Autodesk Inventor part; units mm, degrees
(part 2 of 2)
  spline S28 degree 3 poles (-3.689, -11.9815) (-3.6809, -11.9574) (-3.6638, -11.908) (-3.6373, -11.8352) (-3.6101, -11.7647) (-3.5836, -11.699) (-3.5531, -11.629) (-3.5301, -11.5735) (-3.5094, -11.5336) (-3.5004, -11.5147) (-3.492, -11.4959) (-3.4842, -11.4771) (-3.477, -11.4583) (-3.4704, -11.4394) (-3.4644, -11.4203) (-3.4591, -11.401) (-3.4546, -11.3811) (-3.4508, -11.3607) (-3.4479, -11.3394) (-3.4461, -11.3171) (-3.4456, -11.2935) (-3.4468, -11.2683) (-3.4503, -11.2414) (-3.4567, -11.2125) (-3.4668, -11.1819) (-3.4815, -11.1502) (-3.5016, -11.1183) (-3.5261, -11.0891) (-3.5749, -11.0459) (-3.6488, -10.9917) (-3.7179, -10.9316) (-3.7709, -10.8935) (-3.8047, -10.876) (-3.8402, -10.8634) (-3.8745, -10.8561) (-3.9066, -10.853) (-3.9361, -10.8531) (-3.9632, -10.8557) (-3.988, -10.86) (-4.0109, -10.8657) (-4.0323, -10.8724) (-4.0524, -10.8799) (-4.0715, -10.8881) (-4.0898, -10.8969) (-4.1075, -10.9063) (-4.1248, -10.9164) (-4.1418, -10.9269) (-4.1585, -10.9381) (-4.1751, -10.9499) (-4.1916, -10.9622) (-4.2081, -10.9752) (-4.2425, -11.0042) (-4.2915, -11.0389) (-4.3531, -11.084) (-4.4113, -11.1243) (-4.4741, -11.1664) (-4.5392, -11.2083) (-4.5836, -11.2358) (-4.6054, -11.2491) knots 0 0 0 0 0.034227 0.070321 0.104238 0.13598 0.165545 0.207076 0.216654 0.226052 0.235294 0.244406 0.25342 0.262376 0.27132 0.280307 0.289405 0.298694 0.308273 0.31826 0.328793 0.340032 0.352153 0.365336 0.379732 0.395424 0.412362 0.430317 0.446471 0.5 0.553529 0.569683 0.587638 0.604576 0.620268 0.634664 0.647847 0.659968 0.671207 0.68174 0.691727 0.701306 0.710595 0.719693 0.72868 0.737624 0.74658 0.755594 0.764706 0.773948 0.783346 0.792924 0.834455 0.86402 0.895762 0.929679 0.965773 1 1 1 1
  arc A28 (-3.689, -11.9815) -> (-2.6062, -12.7155) centre (5.7104, 0.7186) ccw
  spline S29 degree 3 poles (-1.5865, -13.2955) (-1.5823, -13.2704) (-1.5731, -13.219) (-1.5583, -13.1429) (-1.5425, -13.069) (-1.5266, -13) (-1.5075, -12.9261) (-1.4934, -12.8677) (-1.4792, -12.8251) (-1.4733, -12.805) (-1.4679, -12.785) (-1.4631, -12.7653) (-1.459, -12.7456) (-1.4554, -12.7259) (-1.4525, -12.7061) (-1.4503, -12.6862) (-1.4489, -12.6659) (-1.4483, -12.6451) (-1.4488, -12.6236) (-1.4505, -12.6013) (-1.4538, -12.5779) (-1.4589, -12.5533) (-1.4666, -12.5272) (-1.4774, -12.4997) (-1.4921, -12.4711) (-1.5116, -12.442) (-1.5365, -12.4136) (-1.5653, -12.3887) (-1.6202, -12.3536) (-1.7017, -12.3116) (-1.7794, -12.263) (-1.8376, -12.2337) (-1.8738, -12.2217) (-1.9108, -12.2149) (-1.9458, -12.213) (-1.978, -12.2149) (-2.0071, -12.2197) (-2.0334, -12.2265) (-2.0573, -12.2346) (-2.0791, -12.2438) (-2.0991, -12.2537) (-2.1178, -12.2643) (-2.1354, -12.2754) (-2.1521, -12.287) (-2.1681, -12.2991) (-2.1836, -12.3117) (-2.1987, -12.3248) (-2.2135, -12.3384) (-2.2281, -12.3526) (-2.2424, -12.3674) (-2.2567, -12.3828) (-2.2861, -12.4168) (-2.3291, -12.4587) (-2.3829, -12.513) (-2.434, -12.5619) (-2.4895, -12.6133) (-2.5473, -12.6649) (-2.5868, -12.699) (-2.6062, -12.7155) knots 0 0 0 0 0.034227 0.070321 0.104238 0.13598 0.165545 0.207076 0.216654 0.226052 0.235294 0.244406 0.25342 0.262376 0.27132 0.280307 0.289405 0.298694 0.308273 0.31826 0.328793 0.340032 0.352153 0.365336 0.379732 0.395424 0.412362 0.430317 0.446471 0.5 0.553529 0.569683 0.587638 0.604576 0.620268 0.634664 0.647847 0.659968 0.671207 0.68174 0.691727 0.701306 0.710595 0.719693 0.72868 0.737624 0.74658 0.755594 0.764706 0.773948 0.783346 0.792924 0.834455 0.86402 0.895762 0.929679 0.965773 1 1 1 1
  arc A29 (-1.5865, -13.2955) -> (-0.4023, -13.8511) centre (5.7104, 0.7186) ccw
  spline S30 degree 3 poles (0.6956, -14.2644) (0.6959, -14.239) (0.6968, -14.1868) (0.6996, -14.1094) (0.7036, -14.0339) (0.7085, -13.9633) (0.7159, -13.8872) (0.7206, -13.8274) (0.728, -13.783) (0.7307, -13.7622) (0.7329, -13.7417) (0.7345, -13.7215) (0.7356, -13.7014) (0.736, -13.6814) (0.7358, -13.6614) (0.7348, -13.6413) (0.733, -13.621) (0.7303, -13.6004) (0.7265, -13.5793) (0.7213, -13.5576) (0.7145, -13.535) (0.7055, -13.5114) (0.6939, -13.4868) (0.6789, -13.4614) (0.6599, -13.4354) (0.6361, -13.4097) (0.6071, -13.3856) (0.5748, -13.3655) (0.515, -13.3394) (0.428, -13.3107) (0.3436, -13.2749) (0.2815, -13.255) (0.2439, -13.2488) (0.2062, -13.2479) (0.1714, -13.2515) (0.1399, -13.2584) (0.1119, -13.2677) (0.0869, -13.2785) (0.0647, -13.2903) (0.0446, -13.3028) (0.0264, -13.3157) (0.0096, -13.3291) (-0.006, -13.3428) (-0.0207, -13.3568) (-0.0347, -13.3713) (-0.048, -13.3861) (-0.0609, -13.4015) (-0.0734, -13.4173) (-0.0855, -13.4336) (-0.0974, -13.4504) (-0.1091, -13.4678) (-0.1328, -13.506) (-0.1687, -13.5542) (-0.2133, -13.6161) (-0.2562, -13.6724) (-0.303, -13.7319) (-0.352, -13.7919) (-0.3857, -13.8318) (-0.4023, -13.8511) knots 0 0 0 0 0.034227 0.070321 0.104238 0.13598 0.165545 0.207076 0.216654 0.226052 0.235294 0.244406 0.25342 0.262376 0.27132 0.280307 0.289405 0.298694 0.308273 0.31826 0.328793 0.340032 0.352153 0.365336 0.379732 0.395424 0.412362 0.430317 0.446471 0.5 0.553529 0.569683 0.587638 0.604576 0.620268 0.634664 0.647847 0.659968 0.671207 0.68174 0.691727 0.701306 0.710595 0.719693 0.72868 0.737624 0.74658 0.755594 0.764706 0.773948 0.783346 0.792924 0.834455 0.86402 0.895762 0.929679 0.965773 1 1 1 1
  arc A30 (0.6956, -14.2644) -> (1.9522, -14.6279) centre (5.7104, 0.7186) ccw
  spline S31 degree 3 poles (3.1012, -14.8645) (3.0975, -14.8393) (3.0903, -14.7875) (3.0809, -14.7107) (3.0731, -14.6355) (3.0669, -14.565) (3.0622, -14.4887) (3.0576, -14.4289) (3.0579, -14.3839) (3.0573, -14.3629) (3.0563, -14.3423) (3.0547, -14.3221) (3.0526, -14.3021) (3.0499, -14.2822) (3.0465, -14.2625) (3.0425, -14.2429) (3.0375, -14.2231) (3.0316, -14.2032) (3.0246, -14.1829) (3.016, -14.1623) (3.0057, -14.141) (2.9932, -14.1191) (2.9779, -14.0967) (2.9591, -14.0739) (2.9362, -14.0512) (2.9087, -14.0296) (2.8763, -14.0103) (2.8412, -13.9955) (2.7781, -13.979) (2.6877, -13.9643) (2.5988, -13.9421) (2.5343, -13.9323) (2.4962, -13.932) (2.4589, -13.937) (2.425, -13.946) (2.395, -13.9577) (2.3688, -13.9713) (2.3458, -13.9859) (2.3257, -14.001) (2.3078, -14.0165) (2.2918, -14.0321) (2.2773, -14.0479) (2.264, -14.0639) (2.2517, -14.0801) (2.2402, -14.0965) (2.2293, -14.1133) (2.219, -14.1304) (2.2092, -14.148) (2.1997, -14.166) (2.1906, -14.1845) (2.1818, -14.2035) (2.1644, -14.245) (2.1364, -14.2981) (2.102, -14.3663) (2.0685, -14.4286) (2.0316, -14.4947) (1.9926, -14.5616) (1.9655, -14.6063) (1.9522, -14.6279) knots 0 0 0 0 0.034227 0.070321 0.104238 0.13598 0.165545 0.207076 0.216654 0.226052 0.235294 0.244406 0.25342 0.262376 0.27132 0.280307 0.289405 0.298694 0.308273 0.31826 0.328793 0.340032 0.352153 0.365336 0.379732 0.395424 0.412362 0.430317 0.446471 0.5 0.553529 0.569683 0.587638 0.604576 0.620268 0.634664 0.647847 0.659968 0.671207 0.68174 0.691727 0.701306 0.710595 0.719693 0.72868 0.737624 0.74658 0.755594 0.764706 0.773948 0.783346 0.792924 0.834455 0.86402 0.895762 0.929679 0.965773 1 1 1 1
  arc A31 (3.1012, -14.8645) -> (4.3992, -15.0269) centre (5.7104, 0.7186) ccw
  spline S32 degree 3 poles (5.5711, -15.0808) (5.5635, -15.0565) (5.5482, -15.0065) (5.5269, -14.932) (5.5075, -14.859) (5.4903, -14.7903) (5.4738, -14.7157) (5.4598, -14.6574) (5.4531, -14.6129) (5.4493, -14.5923) (5.445, -14.5721) (5.4403, -14.5523) (5.4351, -14.5329) (5.4293, -14.5137) (5.4229, -14.4948) (5.4158, -14.476) (5.4079, -14.4573) (5.3989, -14.4385) (5.3888, -14.4196) (5.3771, -14.4005) (5.3636, -14.3812) (5.3478, -14.3615) (5.3292, -14.3417) (5.307, -14.3221) (5.2809, -14.3033) (5.2503, -14.2863) (5.2153, -14.2723) (5.1783, -14.2631) (5.1134, -14.2568) (5.0218, -14.2564) (4.9305, -14.2484) (4.8653, -14.2487) (4.8277, -14.2545) (4.7915, -14.2652) (4.7595, -14.2794) (4.7317, -14.2957) (4.7079, -14.3132) (4.6875, -14.3312) (4.67, -14.3493) (4.6548, -14.3673) (4.6414, -14.3853) (4.6296, -14.4032) (4.6189, -14.421) (4.6093, -14.4389) (4.6005, -14.457) (4.5924, -14.4753) (4.5849, -14.4938) (4.5779, -14.5127) (4.5714, -14.5319) (4.5653, -14.5517) (4.5596, -14.5718) (4.5488, -14.6155) (4.5296, -14.6723) (4.5063, -14.7451) (4.4829, -14.8119) (4.4568, -14.8828) (4.4287, -14.955) (4.409, -15.0034) (4.3992, -15.0269) knots 0 0 0 0 0.034227 0.070321 0.104238 0.13598 0.165545 0.207076 0.216654 0.226052 0.235294 0.244406 0.25342 0.262376 0.27132 0.280307 0.289405 0.298694 0.308273 0.31826 0.328793 0.340032 0.352153 0.365336 0.379732 0.395424 0.412362 0.430317 0.446471 0.5 0.553529 0.569683 0.587638 0.604576 0.620268 0.634664 0.647847 0.659968 0.671207 0.68174 0.691727 0.701306 0.710595 0.719693 0.72868 0.737624 0.74658 0.755594 0.764706 0.773948 0.783346 0.792924 0.834455 0.86402 0.895762 0.929679 0.965773 1 1 1 1
  arc A32 (5.5711, -15.0808) -> (6.8785, -15.0381) centre (5.7104, 0.7186) ccw
  spline S33 degree 3 poles (8.0444, -14.908) (8.0331, -14.8853) (8.0102, -14.8383) (7.9775, -14.7681) (7.9468, -14.6989) (7.9192, -14.6338) (7.8912, -14.5627) (7.8682, -14.5073) (7.8547, -14.4644) (7.8476, -14.4446) (7.8403, -14.4254) (7.8325, -14.4066) (7.8243, -14.3882) (7.8156, -14.3702) (7.8064, -14.3525) (7.7964, -14.335) (7.7856, -14.3178) (7.7738, -14.3006) (7.7609, -14.2836) (7.7464, -14.2665) (7.73, -14.2495) (7.7113, -14.2326) (7.6898, -14.216) (7.6649, -14.2001) (7.6361, -14.1856) (7.6033, -14.1735) (7.5665, -14.1652) (7.5285, -14.1619) (7.4634, -14.1658) (7.3729, -14.1798) (7.2815, -14.1861) (7.2171, -14.1967) (7.1808, -14.2082) (7.1468, -14.2244) (7.1174, -14.2435) (7.0925, -14.2639) (7.0717, -14.2849) (7.0544, -14.3059) (7.0399, -14.3265) (7.0277, -14.3467) (7.0173, -14.3665) (7.0084, -14.3861) (7.0007, -14.4054) (6.994, -14.4246) (6.9882, -14.4438) (6.983, -14.4631) (6.9785, -14.4826) (6.9746, -14.5023) (6.9711, -14.5224) (6.9682, -14.5428) (6.9657, -14.5636) (6.9619, -14.6084) (6.9518, -14.6676) (6.9402, -14.7431) (6.9275, -14.8127) (6.9129, -14.8869) (6.8964, -14.9626) (6.8845, -15.0134) (6.8785, -15.0381) knots 0 0 0 0 0.034227 0.070321 0.104238 0.13598 0.165545 0.207076 0.216654 0.226052 0.235294 0.244406 0.25342 0.262376 0.27132 0.280307 0.289405 0.298694 0.308273 0.31826 0.328793 0.340032 0.352153 0.365336 0.379732 0.395424 0.412362 0.430317 0.446471 0.5 0.553529 0.569683 0.587638 0.604576 0.620268 0.634664 0.647847 0.659968 0.671207 0.68174 0.691727 0.701306 0.710595 0.719693 0.72868 0.737624 0.74658 0.755594 0.764706 0.773948 0.783346 0.792924 0.834455 0.86402 0.895762 0.929679 0.965773 1 1 1 1
  arc A33 (8.0444, -14.908) -> (9.329, -14.6614) centre (5.7104, 0.7186) ccw
  spline S34 degree 3 poles (10.4602, -14.3505) (10.4454, -14.3298) (10.4155, -14.287) (10.3722, -14.2227) (10.3311, -14.1593) (10.2936, -14.0993) (10.2548, -14.0334) (10.2235, -13.9823) (10.2034, -13.942) (10.1934, -13.9236) (10.1831, -13.9057) (10.1725, -13.8884) (10.1615, -13.8715) (10.1501, -13.8551) (10.1382, -13.839) (10.1256, -13.8234) (10.1123, -13.808) (10.098, -13.7929) (10.0825, -13.7781) (10.0655, -13.7635) (10.0467, -13.7493) (10.0256, -13.7355) (10.0017, -13.7224) (9.9746, -13.7106) (9.944, -13.7008) (9.9096, -13.6941) (9.872, -13.6916) (9.834, -13.6943) (9.7703, -13.7083) (9.683, -13.7363) (9.5938, -13.7568) (9.5318, -13.7773) (9.4978, -13.7944) (9.4667, -13.8158) (9.4407, -13.8391) (9.4193, -13.8633) (9.4021, -13.8872) (9.3882, -13.9106) (9.3771, -13.9333) (9.3682, -13.9552) (9.3611, -13.9764) (9.3554, -13.997) (9.3508, -14.0173) (9.3471, -14.0373) (9.3444, -14.0572) (9.3423, -14.0771) (9.3409, -14.097) (9.3401, -14.1172) (9.3398, -14.1375) (9.3401, -14.1581) (9.3409, -14.1791) (9.3442, -14.2239) (9.3434, -14.2839) (9.3438, -14.3603) (9.3422, -14.4311) (9.3393, -14.5066) (9.3349, -14.584) (9.3311, -14.6361) (9.329, -14.6614) knots 0 0 0 0 0.034227 0.070321 0.104238 0.13598 0.165545 0.207076 0.216654 0.226052 0.235294 0.244406 0.25342 0.262376 0.27132 0.280307 0.289405 0.298694 0.308273 0.31826 0.328793 0.340032 0.352153 0.365336 0.379732 0.395424 0.412362 0.430317 0.446471 0.5 0.553529 0.569683 0.587638 0.604576 0.620268 0.634664 0.647847 0.659968 0.671207 0.68174 0.691727 0.701306 0.710595 0.719693 0.72868 0.737624 0.74658 0.755594 0.764706 0.773948 0.783346 0.792924 0.834455 0.86402 0.895762 0.929679 0.965773 1 1 1 1
  arc A34 (10.4602, -14.3505) -> (11.6904, -13.906) centre (5.7104, 0.7186) ccw
  spline S35 degree 3 poles (12.759, -13.422) (12.7412, -13.4038) (12.705, -13.3662) (12.6522, -13.3095) (12.6017, -13.2533) (12.5552, -13.1999) (12.5066, -13.1409) (12.4677, -13.0952) (12.4415, -13.0587) (12.4287, -13.0421) (12.4158, -13.026) (12.4026, -13.0105) (12.3891, -12.9956) (12.3753, -12.9811) (12.361, -12.9672) (12.3461, -12.9536) (12.3306, -12.9406) (12.3141, -12.9279) (12.2964, -12.9157) (12.2774, -12.9039) (12.2566, -12.8928) (12.2336, -12.8825) (12.208, -12.8733) (12.1794, -12.8659) (12.1475, -12.861) (12.1125, -12.8597) (12.075, -12.8631) (12.0379, -12.8718) (11.9772, -12.8956) (11.8954, -12.9368) (11.8104, -12.9711) (11.7525, -13.001) (11.7215, -13.0232) (11.6942, -13.0492) (11.6721, -13.0764) (11.6547, -13.1035) (11.6415, -13.1299) (11.6315, -13.1552) (11.6241, -13.1793) (11.6187, -13.2023) (11.615, -13.2243) (11.6125, -13.2457) (11.6112, -13.2664) (11.6107, -13.2867) (11.6111, -13.3068) (11.6121, -13.3268) (11.6139, -13.3467) (11.6162, -13.3667) (11.6192, -13.3868) (11.6227, -13.4071) (11.6267, -13.4277) (11.637, -13.4715) (11.6456, -13.5309) (11.6579, -13.6063) (11.6674, -13.6764) (11.6764, -13.7515) (11.6841, -13.8286) (11.6885, -13.8806) (11.6904, -13.906) knots 0 0 0 0 0.034227 0.070321 0.104238 0.13598 0.165545 0.207076 0.216654 0.226052 0.235294 0.244406 0.25342 0.262376 0.27132 0.280307 0.289405 0.298694 0.308273 0.31826 0.328793 0.340032 0.352153 0.365336 0.379732 0.395424 0.412362 0.430317 0.446471 0.5 0.553529 0.569683 0.587638 0.604576 0.620268 0.634664 0.647847 0.659968 0.671207 0.68174 0.691727 0.701306 0.710595 0.719693 0.72868 0.737624 0.74658 0.755594 0.764706 0.773948 0.783346 0.792924 0.834455 0.86402 0.895762 0.929679 0.965773 1 1 1 1
  arc A35 (12.759, -13.422) -> (13.9046, -12.7904) centre (5.7104, 0.7186) ccw
  spline S36 degree 3 poles (14.8843, -12.1452) (14.8639, -12.1301) (14.8222, -12.0986) (14.7612, -12.0509) (14.7025, -12.0032) (14.6483, -11.9577) (14.5911, -11.9071) (14.5454, -11.8681) (14.5139, -11.836) (14.4987, -11.8217) (14.4834, -11.8078) (14.4679, -11.7946) (14.4523, -11.7819) (14.4363, -11.7698) (14.42, -11.7583) (14.4033, -11.7473) (14.3858, -11.7368) (14.3675, -11.7268) (14.3482, -11.7175) (14.3276, -11.7089) (14.3053, -11.7012) (14.2809, -11.6946) (14.2542, -11.6895) (14.2248, -11.6867) (14.1926, -11.6868) (14.1578, -11.691) (14.1213, -11.7003) (14.086, -11.7146) (14.0298, -11.7476) (13.9554, -11.8012) (13.8769, -11.8483) (13.8243, -11.8869) (13.7972, -11.9137) (13.7743, -11.9436) (13.7567, -11.9739) (13.7438, -12.0034) (13.7348, -12.0316) (13.7289, -12.0581) (13.7254, -12.0831) (13.7237, -12.1066) (13.7234, -12.129) (13.7243, -12.1504) (13.7262, -12.1711) (13.729, -12.1913) (13.7325, -12.2111) (13.7367, -12.2306) (13.7415, -12.25) (13.7469, -12.2694) (13.753, -12.2888) (13.7597, -12.3083) (13.7669, -12.328) (13.7838, -12.3697) (13.8017, -12.427) (13.8256, -12.4995) (13.8459, -12.5673) (13.8665, -12.6401) (13.8863, -12.715) (13.8987, -12.7657) (13.9046, -12.7904) knots 0 0 0 0 0.034227 0.070321 0.104238 0.13598 0.165545 0.207076 0.216654 0.226052 0.235294 0.244406 0.25342 0.262376 0.27132 0.280307 0.289405 0.298694 0.308273 0.31826 0.328793 0.340032 0.352153 0.365336 0.379732 0.395424 0.412362 0.430317 0.446471 0.5 0.553529 0.569683 0.587638 0.604576 0.620268 0.634664 0.647847 0.659968 0.671207 0.68174 0.691727 0.701306 0.710595 0.719693 0.72868 0.737624 0.74658 0.755594 0.764706 0.773948 0.783346 0.792924 0.834455 0.86402 0.895762 0.929679 0.965773 1 1 1 1
  arc A36 (14.8843, -12.1452) -> (15.917, -11.3423) centre (5.7104, 0.7186) ccw
  spline S37 degree 3 poles (16.7837, -10.5517) (16.7612, -10.5399) (16.7151, -10.5154) (16.6473, -10.4778) (16.5819, -10.4399) (16.5213, -10.4035) (16.4568, -10.3624) (16.4057, -10.331) (16.3695, -10.3043) (16.3522, -10.2925) (16.3349, -10.2812) (16.3176, -10.2706) (16.3002, -10.2605) (16.2825, -10.251) (16.2646, -10.2422) (16.2463, -10.2339) (16.2275, -10.2263) (16.2079, -10.2193) (16.1873, -10.2132) (16.1656, -10.2079) (16.1423, -10.2037) (16.1173, -10.201) (16.0901, -10.2002) (16.0606, -10.202) (16.0288, -10.2072) (15.9951, -10.2168) (15.9605, -10.2316) (15.9279, -10.2513) (15.8775, -10.2927) (15.8124, -10.3572) (15.7422, -10.4161) (15.6964, -10.4625) (15.6738, -10.4931) (15.6558, -10.5263) (15.6432, -10.5589) (15.6351, -10.5901) (15.6306, -10.6193) (15.6289, -10.6464) (15.6293, -10.6716) (15.6313, -10.6952) (15.6346, -10.7173) (15.6388, -10.7383) (15.644, -10.7585) (15.6498, -10.778) (15.6564, -10.797) (15.6636, -10.8156) (15.6714, -10.834) (15.6798, -10.8523) (15.6888, -10.8705) (15.6984, -10.8888) (15.7086, -10.9071) (15.7319, -10.9456) (15.7585, -10.9994) (15.7934, -11.0673) (15.8241, -11.1311) (15.8559, -11.1997) (15.8871, -11.2706) (15.9073, -11.3188) (15.917, -11.3423) knots 0 0 0 0 0.034227 0.070321 0.104238 0.13598 0.165545 0.207076 0.216654 0.226052 0.235294 0.244406 0.25342 0.262376 0.27132 0.280307 0.289405 0.298694 0.308273 0.31826 0.328793 0.340032 0.352153 0.365336 0.379732 0.395424 0.412362 0.430317 0.446471 0.5 0.553529 0.569683 0.587638 0.604576 0.620268 0.634664 0.647847 0.659968 0.671207 0.68174 0.691727 0.701306 0.710595 0.719693 0.72868 0.737624 0.74658 0.755594 0.764706 0.773948 0.783346 0.792924 0.834455 0.86402 0.895762 0.929679 0.965773 1 1 1 1
  arc A37 (16.7837, -10.5517) -> (17.6781, -9.5971) centre (5.7104, 0.7186) ccw
  spline S38 degree 3 poles (18.4105, -8.6807) (18.3864, -8.6726) (18.337, -8.6555) (18.2642, -8.629) (18.1937, -8.6018) (18.128, -8.5754) (18.058, -8.5449) (18.0025, -8.5219) (17.9626, -8.5011) (17.9437, -8.4922) (17.9249, -8.4837) (17.9061, -8.4759) (17.8873, -8.4687) (17.8684, -8.4621) (17.8493, -8.4562) (17.83, -8.4509) (17.8101, -8.4463) (17.7897, -8.4425) (17.7684, -8.4396) (17.7461, -8.4378) (17.7225, -8.4374) (17.6974, -8.4386) (17.6704, -8.4421) (17.6415, -8.4484) (17.611, -8.4585) (17.5792, -8.4732) (17.5473, -8.4933) (17.5181, -8.5179) (17.4749, -8.5667) (17.4207, -8.6406) (17.3606, -8.7097) (17.3225, -8.7626) (17.305, -8.7965) (17.2924, -8.832) (17.2851, -8.8663) (17.282, -8.8983) (17.2821, -8.9279) (17.2847, -8.9549) (17.289, -8.9798) (17.2947, -9.0027) (17.3014, -9.024) (17.3089, -9.0441) (17.3171, -9.0632) (17.3259, -9.0816) (17.3353, -9.0993) (17.3454, -9.1166) (17.356, -9.1335) (17.3671, -9.1503) (17.3789, -9.1669) (17.3913, -9.1834) (17.4042, -9.1999) (17.4332, -9.2342) (17.4679, -9.2832) (17.513, -9.3449) (17.5533, -9.403) (17.5954, -9.4658) (17.6373, -9.531) (17.6648, -9.5754) (17.6781, -9.5971) knots 0 0 0 0 0.034227 0.070321 0.104238 0.13598 0.165545 0.207076 0.216654 0.226052 0.235294 0.244406 0.25342 0.262376 0.27132 0.280307 0.289405 0.298694 0.308273 0.31826 0.328793 0.340032 0.352153 0.365336 0.379732 0.395424 0.412362 0.430317 0.446471 0.5 0.553529 0.569683 0.587638 0.604576 0.620268 0.634664 0.647847 0.659968 0.671207 0.68174 0.691727 0.701306 0.710595 0.719693 0.72868 0.737624 0.74658 0.755594 0.764706 0.773948 0.783346 0.792924 0.834455 0.86402 0.895762 0.929679 0.965773 1 1 1 1
  arc A38 (18.4105, -8.6807) -> (19.1445, -7.598) centre (5.7104, 0.7186) ccw
  spline S39 degree 3 poles (19.7245, -6.5783) (19.6994, -6.574) (19.648, -6.5649) (19.5719, -6.5501) (19.498, -6.5343) (19.429, -6.5184) (19.3551, -6.4993) (19.2967, -6.4852) (19.2541, -6.471) (19.234, -6.4651) (19.2141, -6.4597) (19.1943, -6.4549) (19.1746, -6.4507) (19.1549, -6.4472) (19.1351, -6.4443) (19.1152, -6.4421) (19.0949, -6.4407) (19.0741, -6.4401) (19.0527, -6.4406) (19.0303, -6.4423) (19.007, -6.4455) (18.9823, -6.4507) (18.9562, -6.4583) (18.9287, -6.4691) (18.9001, -6.4839) (18.871, -6.5034) (18.8426, -6.5282) (18.8177, -6.557) (18.7826, -6.612) (18.7406, -6.6934) (18.692, -6.7711) (18.6628, -6.8294) (18.6508, -6.8655) (18.6439, -6.9026) (18.642, -6.9376) (18.6439, -6.9697) (18.6487, -6.9989) (18.6555, -7.0252) (18.6636, -7.049) (18.6728, -7.0708) (18.6828, -7.0909) (18.6933, -7.1095) (18.7044, -7.1271) (18.716, -7.1438) (18.7281, -7.1599) (18.7407, -7.1754) (18.7538, -7.1905) (18.7674, -7.2053) (18.7817, -7.2198) (18.7965, -7.2342) (18.8118, -7.2485) (18.8459, -7.2779) (18.8878, -7.3208) (18.942, -7.3746) (18.9909, -7.4258) (19.0423, -7.4812) (19.0939, -7.539) (19.128, -7.5786) (19.1445, -7.598) knots 0 0 0 0 0.034227 0.070321 0.104238 0.13598 0.165545 0.207076 0.216654 0.226052 0.235294 0.244406 0.25342 0.262376 0.27132 0.280307 0.289405 0.298694 0.308273 0.31826 0.328793 0.340032 0.352153 0.365336 0.379732 0.395424 0.412362 0.430317 0.446471 0.5 0.553529 0.569683 0.587638 0.604576 0.620268 0.634664 0.647847 0.659968 0.671207 0.68174 0.691727 0.701306 0.710595 0.719693 0.72868 0.737624 0.74658 0.755594 0.764706 0.773948 0.783346 0.792924 0.834455 0.86402 0.895762 0.929679 0.965773 1 1 1 1
  arc A39 (19.7245, -6.5783) -> (20.2801, -5.394) centre (5.7104, 0.7186) ccw
  circle A40 centre (9.6659, 7.6723) radius 2.35
  circle A41 centre (-1.2433, 4.6741) radius 2.35
  circle A42 centre (1.7549, -6.2351) radius 2.35
  circle A43 centre (5.7104, 0.7186) radius 4.5
  circle A44 centre (12.6641, -3.2369) radius 2.35
  circle A45 centre (5.7104, 0.7186) radius 4.5
  point P0 (0, 0)
  constraints: 1 centre point, 1 coincident, 1 concentric
extrude "Выдавливание2" add sketch "Эскиз2" along normal blind 6.35 contours A43
